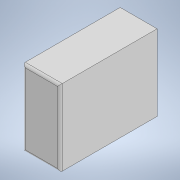
# Autodesk Inventor part: block1
Saved by Autodesk Inventor 2020.1 (Build 241239000, 239)
## iProperties
Created: 2020-01-22
Part Number: block1
Material: Generic
Document SubType Name: Modeling
Designer: Ali
Density: 1 g/cm^3
Appearance: Default
Author: Ali
Autodesk Inventor part; units mm, degrees
ref_plane "YZ Plane" through (0, 0, 0) normal (1, 0, 0) x (0, 1, 0)
ref_plane "XZ Plane" through (0, 0, 0) normal (0, 1, 0) x (-1, 0, 0)
ref_plane "XY Plane" through (0, 0, 0) normal (0, 0, 1) x (1, 0, 0)
sketch "Sketch1" plane through (0, 0, 0) normal (0, 0, 1) x (1, 0, 0)
  line L0 (0, 0) -> (3.8, 0)
  line L1 (3.8, 0) -> (3.8, -7.8)
  line L2 (3.8, -7.8) -> (0, -7.8)
  line L3 (0, -7.8) -> (0, 0)
  dimension "d0" = 3.8
  dimension "d1" = 7.8
  constraints: 8 end point, 2 parallel, 1 horizontal, 1 perpendicular
  measures "d0" distance of L0.start L0.end
  measures "d1" distance of L2.end L0.start
extrude "Extrusion1" add sketch "Sketch1" against normal blind 10
fillet "Fillet1" radius 0.25 4 edges at (1.9, 0, 0) (0, -3.9, 0) (3.8, -3.9, 0) (1.9, -7.8, 0)
equation "\"d0\" = BL_width"
equation "\"d1\" = BL_length"
equation "\"d2\" = BL_depth"
equation "\"d4\" = W_filletRadius"
equation "\"Wheel_Related_W_\" = 0"
equation "\"W_innerDepth\" = 4"
equation "\"W_wallThickness\" = 2"
equation "\"W_holesClearance\" = 0.3"
equation "\"W_outerGearHoleDiameter\" = 5.3"
equation "\"W_innerGearHoleDiameter\" = 10.1"
equation "\"TempSpotReserved7\" = 0"
equation "\"TempSpotReserved8\" = 0"
equation "\"TempSpotReserved9\" = 0"
equation "\"TempSpotReserved10\" = 0"
equation "\"Inner_Gear_Related_IG_\" = 0"
equation "\"IG_shaftDiameter\" = 7.5"
equation "\"IG_shaftLength\" = 15"
equation "\"IG_gearThickness\" = 2"
equation "\"IG_ratioToOuterGear\" = 0.75"
equation "\"IG_skirtThickness\" = 2"
equation "\"IG_extentionLength\" = 18.33333"
equation "\"IG_extentionThickness\" = 3"
equation "\"IG_slitWidth\" = 4"
equation "\"IG_slitlength\" = 8"
equation "\"Outer_Gear_Related_OG_\" = 0"
equation "\"OG_distanceFromCenter\" = 23.33333"
equation "\"OG_shaftDiameter\" = 5"
equation "\"OG_gearDiameter\" = 26.66667"
equation "\"OG_shaftLength\" = 7"
equation "\"OG_gearThickness\" = 2"
equation "\"OG_skirtOffset\" = 1"
equation "\"OG_skirtThickness\" = 1"
equation "\"TempSpotReserved29\" = 0"
equation "\"TempSpotReserved30\" = 0"
equation "\"Leg_Extensions_Related_LE_\" = 0"
equation "\"LE_baseDiameter\" = 5"
equation "\"LE_maxLength\" = 24.6522"
equation "\"LE_thickness\" = 2.5"
equation "\"LE_offsetAboveOuterGear\" = 0"
equation "\"TempSpotReserved35\" = 0"
equation "\"TempSpotReserved36\" = 0"
equation "\"TempSpotReserved37\" = 0"
equation "\"TempSpotReserved38\" = 0"
equation "\"TempSpotReserved39\" = 0"
equation "\"TempSpotReserved40\" = 0"
equation "\"Bearing_Related_B_\" = 0"
equation "\"B_bearingThickness\" = 1"
equation "\"TempSpotReserved42\" = 0"
equation "\"TempSpotReserved43\" = 0"
equation "\"TempSpotReserved44\" = 0"
equation "\"TempSpotReserved45\" = 0"
equation "\"TempSpotReserved46\" = 0"
equation "\"TempSpotReserved47\" = 0"
equation "\"TempSpotReserved48\" = 0"
equation "\"TempSpotReserved49\" = 0"
equation "\"TempSpotReserved50\" = 0"
equation "\"IG_slitDistanceFromCenterHole\" = 8"
equation "\"IG_slitClearance\" = 0.2"
equation "\"Reserved_10\" = 0"
equation "\"Reserved_9\" = 0"
equation "\"Reserved_11\" = 0"
equation "\"Reserved_12\" = 0"
equation "\"Reserved_8\" = 0"
equation "\"Reserved_7\" = 0"
equation "\"Reserved_26\" = 0"
equation "\"Reserved_20\" = 0"
equation "\"Reserved_22\" = 0"
equation "\"Reserved_23\" = 0"
equation "\"Reserved_25\" = 0"
equation "\"Reserved_24\" = 0"
equation "\"Reserved_21\" = 0"
equation "\"Reserved_19\" = 0"
equation "\"Reserved_27\" = 0"
equation "\"Reserved_14\" = 0"
equation "\"Reserved_15\" = 0"
equation "\"Reserved_16\" = 0"
equation "\"Reserved_13\" = 0"
equation "\"Reserved_17\" = 0"
equation "\"Reserved_18\" = 0"
equation "\"Bearing_Related_BR_\" = 0"
equation "\"BR_bearingThickness\" = 1"
equation "\"Block_Related_BL_\" = 0"
equation "\"BL_width\" = 3.8"
equation "\"BL_length\" = 7.8"
equation "\"BL_depth\" = 10"
equation "\"W_filletRadius\" = 0.25"
equation "\"W_extrutsionTaperAngle\" = 2deg"
equation "\"OG_protrudeDistance\" = 3"
body "Solid1"
